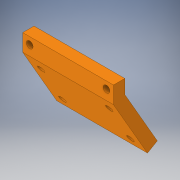
# Autodesk Inventor part: PaddleCollection2.1AngleBracket
Saved by Autodesk Inventor 2019 (Build 230136000, 136)
## iProperties
Created: 2018-10-30
Part Number: PaddleCollection2.1AngleBracket
Material: Nylon 6/6
Document SubType Name: Modeling
Designer: User
Density: 1.13 g/cm^3
Appearance: Orange
Author: User
Autodesk Inventor part; units mm, degrees
ref_plane "YZ Plane" through (0, 0, 0) normal (1, 0, 0) x (0, 1, 0)
ref_plane "XZ Plane" through (0, 0, 0) normal (0, 1, 0) x (-1, 0, 0)
ref_plane "XY Plane" through (0, 0, 0) normal (0, 0, 1) x (1, 0, 0)
sketch "Sketch1" plane through (0, 0, 0) normal (1, 0, 0) x (0, 1, 0)
  line L0 (0, 0) -> (-9.525, 0)
  line L1 (-9.525, 0) -> (-9.525, -6.35)
  line L2 (-9.525, -6.35) -> (0, -6.35)
  line L3 (0, -6.35) -> (0, 0)
  dimension "d0" = 9.525
  dimension "d1" = 6.35
  constraints: 8 end point, 2 parallel, 1 horizontal, 1 perpendicular
  measures "d0" distance of L2.end L1.end
  measures "d1" distance of L1.end L0.end
extrude "Extrusion1" add sketch "Sketch1" along normal blind 50.8
ref_plane "Work Plane1" through (0, -9.525, 0) normal (0, -0.8660254, -0.5) x (1, 0, 0)
sketch "Sketch2" plane through (0, -9.525, 0) normal (0, -0.8660254, -0.5) x (1, 0, 0)
  line L0 (0, 0) -> (50.8, 0) projected
  line L1 (0, -5.4993) -> (0, -10.2618) projected
  line L2 (50.8, 0) -> (0, 0)
  line L3 (0, 0) -> (0, -6.35)
  line L4 (0, -6.35) -> (50.8, -6.35)
  line L5 (50.8, -6.35) -> (50.8, 0)
  point P0 (0, -4.7625)
  dimension "d5" = 6.35
  constraints: 8 end point, 2 parallel, 1 horizontal, 1 perpendicular, 1 point on line
  measures "d5" distance of L3.end L2.end
extrude "Extrusion2" add sketch "Sketch2" along normal blind 38.1
sketch "Sketch3" plane through (50.8, 0, -6.35) normal (0, 0, -1) x (-1, 0, 0)
  line L0 (50.8, 0) -> (0, 0) projected
  line L1 (0, -7.8235) -> (0, 0) projected
  point P0 (3.9118, -3.9118)
  point P1 (46.8882, -3.9118)
  dimension "d8" = 3.9118
  dimension "d9" = 7.8235
  dimension "d10" = 3.9118
  dimension "d11" = 3.9118
  dimension "d12" = 3.9118
  measures "d8" distance from line of point (3.912, -3.912) L0
  measures "d9" distance of L1.start L0.end
  measures "d10" distance from line of L0 point (46.888, -3.912)
  measures "d11" distance from line of L1 point (3.912, -3.912)
  measures "d12" horizontal distance of L0.start point (46.888, -3.912)
hole "Hole1" at (46.8882, -3.9118, -6.35) at (3.9118, -3.9118, -6.35) direction (0, 0, 1) diameter 3.81 end through all
sketch "Sketch4" plane through (50.8, -7.8235, -6.35) normal (0, 0.5, -0.8660254) x (-1, 0, 0)
  line L0 (0, 0) -> (50.8, 0) projected
  line L1 (0, 0) -> (0, -36.3985) projected
  line L2 (50.8, -36.3985) -> (0, -36.3985) projected
  line L3 (50.8, 0) -> (50.8, -36.3985) projected
  point P0 (50.8, 9.9504)
  point P1 (44.45, -6.35)
  point P2 (44.45, -30.0485)
  point P3 (6.35, -6.35)
  point P4 (6.35, -30.0485)
  dimension "d20" = 6.35
  dimension "d21" = 6.35
  dimension "d22" = 6.35
  dimension "d23" = 6.35
  dimension "d24" = 6.35
  dimension "d25" = 6.35
  dimension "d26" = 6.35
  dimension "d27" = 6.35
  measures "d20" distance from line of L3 point (44.45, -6.35)
  measures "d21" distance from line of L0 point (44.45, -6.35)
  measures "d22" distance from line of L3 point (44.45, -30.049)
  measures "d23" distance from line of L2 point (44.45, -30.049)
  measures "d24" distance from line of L0 point (6.35, -6.35)
  measures "d25" distance from line of L1 point (6.35, -6.35)
  measures "d26" distance from line of L1 point (6.35, -30.049)
  measures "d27" distance from line of L2 point (6.35, -30.049)
hole "Hole2" at (6.35, -13.3228, -9.525) at (6.35, -33.8463, -21.3743) at (44.45, -13.3228, -9.525) at (44.45, -33.8463, -21.3743) direction (0, -0.5, 0.8660254) diameter 3.81 end through all
equation "\"d8\" = 0.5 * d9"
equation "\"d10\" = d8"
equation "\"d11\" = d8"
equation "\"d12\" = d8"
equation "\"d21\" = d20"
equation "\"d22\" = d20"
equation "\"d23\" = d20"
equation "\"d24\" = d20"
equation "\"d25\" = d20"
equation "\"d26\" = d20"
equation "\"d27\" = d20"
body "Solid1"
